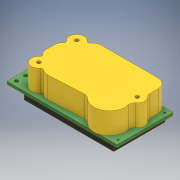
# Autodesk Inventor part: 66-0008
Saved by Autodesk Inventor 2018 (Build 220112000, 112)
## iProperties
Created: 2020-01-31
Part Number: 66-0008
Material: ABS Plastic
Document SubType Name: Modeling
Designer: Bradley
Density: 1.06 g/cm^3
Appearance: Glossy - Gold
Author: Bradley
Autodesk Inventor part; units mm, degrees
ref_plane "YZ Plane" through (0, 0, 0) normal (1, 0, 0) x (0, 1, 0)
ref_plane "XZ Plane" through (0, 0, 0) normal (0, 1, 0) x (-1, 0, 0)
ref_plane "XY Plane" through (0, 0, 0) normal (0, 0, 1) x (1, 0, 0)
sketch "Sketch1" plane through (0, 0, 0) normal (0, 0, 1) x (1, 0, 0)
  line L0 (-14.985, -7.62) -> (14.985, -7.62)
  line L1 (14.985, -7.62) -> (14.985, 7.62)
  line L2 (14.985, 7.62) -> (-14.985, 7.62)
  line L3 (-14.985, 7.62) -> (-14.985, -7.62)
  line L4 (-14.985, -7.62) -> (14.985, 7.62) construction
  line L5 (14.985, -7.62) -> (-14.985, 7.62) construction
  circle A0 centre (-13.715, 6.35) radius 0.5
  circle A1 centre (-13.715, 3.81) radius 0.5
  circle A2 centre (-13.715, 1.27) radius 0.5
  circle A3 centre (-13.715, -1.27) radius 0.5
  circle A4 centre (-13.715, -3.81) radius 0.5
  circle A5 centre (-13.715, -6.35) radius 0.5
  circle A6 centre (13.975, 6.35) radius 0.3
  circle A7 centre (13.975, -6.35) radius 0.3
  point P0 (0, 0)
  dimension "d0" = 29.97
  dimension "d1" = 15.24
  dimension "d2" = 1
  dimension "d3" = 1.27
  dimension "d4" = 1.27
  dimension "d7" = 2.54
  dimension "d12" = 0.6
  dimension "d13" = 28.96
  constraints: 12 end point, 8 centre point, 2 horizontal alignment, 2 midpoint, 2 parallel, 1 equal radius, 1 horizontal, 1 perpendicular, 1 vertical, 1 vertical alignment, 10 other
  measures "d0" distance of L2.end L1.end
  measures "d1" distance of L2.end L0.start
  measures "d2" diameter of A0
  measures "d3" distance from line of L3 A0.centre
  measures "d4" distance from line of A0.centre L2
  measures "d7" distance of A0.centre A1.centre
  measures "d12" diameter of A6
  measures "d13" distance from line of A6.centre L3
extrude "Extrusion1" add sketch "Sketch1" along normal mid plane 0.79
sketch "Sketch2" plane through (0, 0, -0.395) normal (0, 0, -1) x (-1, 0, 0)
  circle A0 centre (13.715, -6.35) radius 0.5 projected
  circle A1 centre (13.715, -3.81) radius 0.5 projected
  circle A2 centre (13.715, -1.27) radius 0.5 projected
  circle A3 centre (13.715, 1.27) radius 0.5 projected
  circle A4 centre (13.715, 3.81) radius 0.5 projected
  circle A5 centre (13.715, 6.35) radius 0.5 projected
  circle A6 centre (-13.975, -6.35) radius 0.3 projected
  circle A7 centre (-13.975, 6.35) radius 0.3 projected
  line L0 (-14.985, -7.62) -> (14.985, -7.62) projected
  line L1 (14.985, -7.62) -> (14.985, 7.62) projected
  line L2 (14.985, 7.62) -> (-14.985, 7.62) projected
  line L3 (-14.985, 7.62) -> (-14.985, -7.62) projected
  line L4 (-13.485, 7) -> (10.985, 7)
  line L5 (10.985, 7) -> (10.985, -7)
  line L6 (10.985, -7) -> (-13.485, -7)
  line L7 (-13.485, -7) -> (-13.485, 7)
  point P0 (0, 0)
  point P1 (10.985, 0)
  dimension "d16" = 14
  dimension "d17" = 4
  dimension "d18" = 1.5
  constraints: 8 end point, 2 parallel, 1 horizontal, 1 horizontal alignment, 1 midpoint, 1 perpendicular
  measures "d16" distance of L4.end L5.end
  measures "d17" distance between parallel lines of L1 L5
  measures "d18" distance between parallel lines of L3 L7
extrude "Extrusion2" add sketch "Sketch2" along normal blind 1.95 contours L4 L5 L6 L7
sketch "Sketch3" plane through (0, 0, 0.395) normal (0, 0, 1) x (1, 0, 0)
  circle A0 centre (-13.715, -6.35) radius 0.5 projected
  circle A1 centre (-13.715, -3.81) radius 0.5 projected
  circle A2 centre (-13.715, -1.27) radius 0.5 projected
  circle A3 centre (-13.715, 1.27) radius 0.5 projected
  circle A4 centre (-13.715, 3.81) radius 0.5 projected
  circle A5 centre (-13.715, 6.35) radius 0.5 projected
  circle A6 centre (13.975, -6.35) radius 0.3 projected
  circle A7 centre (13.975, 6.35) radius 0.3 projected
  line L0 (-14.985, -7.62) -> (14.985, -7.62) projected
  line L1 (14.985, -7.62) -> (14.985, 7.62) projected
  line L2 (14.985, 7.62) -> (-14.985, 7.62) projected
  line L3 (-14.985, 7.62) -> (-14.985, -7.62) projected
  line L4 (-14.985, 7.5559) -> (14.985, 7.5559) construction
  line L5 (14.985, 7.5559) -> (14.985, -7.62) construction
  line L6 (14.985, -7.62) -> (-14.985, -7.62) construction
  line L7 (-14.985, -7.62) -> (-14.985, 7.5559) construction
  line L8 (-14.985, 7.62) -> (-14.985, -7.62) projected
  arc A8 (13.285, 3.0475) -> (13.7564, 1.9557) centre (14.785, 3.0475) ccw
  arc A9 (13.5911, -1.0954) -> (13.7564, 1.9557) centre (12.385, 0.5) ccw
  arc A10 (13.5911, -1.0954) -> (13.032, -2.6201) centre (14.4957, -2.292) ccw
  arc A11 (5.9038, -6.579) -> (13.032, -2.6201) centre (8.885, -3.55) ccw
  arc A12 (5.9038, -6.579) -> (4.3962, -6.0072) centre (4.5009, -8.0044) ccw
  line L9 (4.3962, -6.0072) -> (-5.0076, -6.5)
  arc A13 (-6.7728, -5.8952) -> (-5.0076, -6.5) centre (-5.1385, -4.0034) ccw
  arc A14 (-6.7728, -5.8952) -> (-7.6381, -5.9802) centre (-7.165, -6.3493) ccw
  arc A15 (-10.454, -3.18) -> (-7.6381, -5.9802) centre (-9.215, -4.75) ccw
  arc A16 (-10.454, -3.18) -> (-10.454, -2.395) centre (-10.7637, -2.7875) ccw
  arc A17 (-11.215, -0.825) -> (-10.454, -2.395) centre (-9.215, -0.825) ccw
  line L10 (-11.215, -0.825) -> (-11.215, 1.675)
  arc A18 (-10.454, 3.245) -> (-11.215, 1.675) centre (-9.215, 1.675) ccw
  arc A19 (-10.454, 3.245) -> (-10.454, 4.03) centre (-10.7637, 3.6375) ccw
  arc A20 (-7.6381, 6.8302) -> (-10.454, 4.03) centre (-9.215, 5.6) ccw
  arc A21 (-7.6381, 6.8302) -> (-6.6908, 6.8317) centre (-7.165, 7.1993) ccw
  line L11 (13.285, 3.0475) -> (13.285, 5.3)
  arc A22 (13.285, 5.3) -> (10.785, 7.8) centre (10.785, 5.3) ccw
  line L12 (10.785, 7.8) -> (-4.715, 7.8)
  arc A23 (-4.715, 7.8) -> (-6.6908, 6.8317) centre (-4.715, 5.3) ccw
  circle A24 centre (-9.215, 5.6) radius 0.5
  circle A25 centre (-9.215, -4.75) radius 0.5
  circle A26 centre (12.385, 0.5) radius 0.5
  line L13 (8.885, -7.8) -> (8.885, 7.8) construction
  point P0 (0, 0)
  point P1 (8.885, 0)
  dimension "d29" = 7.8
  dimension "d32" = 4.5
  dimension "d33" = 2.5
  dimension "d34" = 26.1
  dimension "d35" = 24.5
  dimension "d36" = 5.6
  dimension "d37" = 4.75
  dimension "d38" = 2
  dimension "d44" = 2.5
  dimension "d46" = 0.5
  dimension "d49" = 2
  dimension "d52" = 0.6
  dimension "d53" = 2.5
  dimension "d54" = 4.5
  dimension "d57" = 2.5
  dimension "d59" = 0.5
  dimension "d61" = 2
  dimension "d64" = 1.5
  dimension "d65" = 1
  dimension "d73" = 20.1
  dimension "d77" = 4.25
  dimension "d78" = 3
  dimension "d80" = 2.5
  dimension "d82" = 6.5
  dimension "d84" = 2
  constraints: 33 point on circle, 20 tangent, 19 centre point, 10 end point, 7 equal radius, 4 coincident, 3 vertical, 3 vertical alignment, 2 perpendicular, 2 point on line, 1 collinear, 1 horizontal alignment, 1 midpoint, 2 other
  measures "d29" distance from line of point (0, 0) L12
  measures "d32" horizontal distance of A5.centre A20.centre
  measures "d33" distance from line of L10 A5.centre
  measures "d34" horizontal distance of A5.centre A9.centre
  measures "d35" distance between parallel lines of L10 L11
  measures "d36" vertical distance of point (0, 0) A20.centre
  measures "d37" vertical distance of point (0, 0) A15.centre
  measures "d38" radius of A20
  measures "d44" distance of L10.start L10.end
  measures "d46" radius of A19
  measures "d49" radius of A18
  measures "d52" radius of A21
  measures "d53" radius of A23
  measures "d54" horizontal distance of A20.centre A23.centre
  measures "d57" radius of A22
  measures "d59" vertical distance of A9.centre point (0, 0)
  measures "d61" radius of A9
  measures "d64" radius of A8
  measures "d65" diameter of A24
  measures "d73" distance between parallel lines of L10 L13
  measures "d77" radius of A11
  measures "d78" angle of L6 L9
  measures "d80" radius of A13
  measures "d82" vertical distance of point (0, 0) L9.end
  measures "d84" radius of A12
extrude "Extrusion3" add sketch "Sketch3" along normal blind 5.87 contours A11 A12 L9 A13 A14 A15 A16 A17 L10 A18 A19 A20 A21 A23 L2 A22 L11 A8 A9 A10 L0 | L0 A11 | A23 L12 A22 L2
equation "\"d4\" = d3"
body "Solid1"
